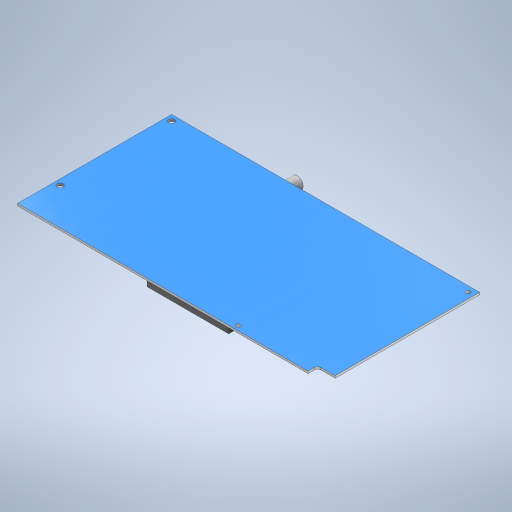
# Autodesk Inventor part: motherboard
Saved by Autodesk Inventor 2024 (Build 280153000, 153)
## iProperties
Created: 2024-09-23
Part Number: motherboard
Material: Generic
Document SubType Name: Modeling
Designer: PC
Density: 1 g/cm^3
Appearance: Default
Author: PC
Autodesk Inventor part; units mm, degrees
ref_plane "YZ Plane" through (0, 0, 0) normal (1, 0, 0) x (0, 1, 0)
ref_plane "XZ Plane" through (0, 0, 0) normal (0, 1, 0) x (-1, 0, 0)
ref_plane "XY Plane" through (0, 0, 0) normal (0, 0, 1) x (1, 0, 0)
sketch "Sketch1" plane through (0, 0, 0) normal (0, 1, 0) x (-1, 0, 0)
  line L0 (12, 0) -> (210, 0)
  line L1 (210, 0) -> (210, -105)
  line L2 (210, -105) -> (0, -105)
  circle A0 centre (4, -101) radius 1.5
  circle A1 centre (206, -101) radius 2
  circle A2 centre (206, -25) radius 2
  circle A3 centre (62.6, -3) radius 1.5
  line L3 (12, 0) -> (12, -4.5)
  line L4 (10, -6.5) -> (0, -6.5)
  arc A4 (10, -6.5) -> (12, -4.5) centre (10, -4.5) ccw
  line L5 (0, -6.5) -> (0, -105)
  point P0 (0, 0)
  point P1 (12, -6.5)
  dimension "d0" = 105
  dimension "d1" = 210
  dimension "d4" = 4
  dimension "d6" = 3
  dimension "d7" = 4
  dimension "d8" = 4
  dimension "d9" = 4
  dimension "d10" = 76
  dimension "d12" = 3
  dimension "d13" = 3
  dimension "d14" = 12
  dimension "d15" = 6.5
  dimension "d16" = 2
  constraints: 12 end point, 5 centre point, 2 point on circle, 2 point on line, 2 tangent, 1 horizontal, 1 parallel, 1 perpendicular, 1 vertical
  measures "d0" distance of L0.end L1.end
  measures "d1" distance of L1.end L2.end
  measures "d4" distance from line of L2 A0.centre
  measures "d6" diameter of A0
  measures "d7" diameter of A1
  measures "d8" distance from line of L1 A1.centre
  measures "d9" diameter of A2
  measures "d10" distance of A1.centre A2.centre
  measures "d12" distance from line of L0 A3.centre
  measures "d13" diameter of A3
  measures "d14" distance of point (12, -6.5) L4.end
  measures "d15" distance of L0.start point (12, -6.5)
  measures "d16" radius of A4
extrude "Extrusion1" add sketch "Sketch1" along normal blind 1.5
sketch "Sketch2" plane through (0, 0, 0) normal (0, -1, 0) x (1, 0, 0)
  line L0 (-126.75, -5) -> (-71.15, -5)
  line L1 (-71.15, -5) -> (-71.15, -9.5)
  line L2 (-71.15, -9.5) -> (-126.75, -9.5)
  line L3 (-126.75, -9.5) -> (-126.75, -5)
  line L4 (-210, -105) -> (-210, 0) projected
  line L5 (0, -6.5) -> (0, -105) projected
  line L6 (-72.7, -8.25) -> (-125.2, -8.25)
  line L7 (-125.2, -8.25) -> (-125.2, -6.25)
  line L8 (-125.2, -6.25) -> (-72.7, -6.25)
  line L9 (-72.7, -6.25) -> (-72.7, -8.25)
  line L10 (-210, 0) -> (-12, 0) projected
  point P0 (0, 0)
  point P1 (-126.75, -7.25)
  point P2 (-72.7, -7.25)
  point P3 (-71.15, -7.25)
  point P4 (-98.95, -6.25)
  point P5 (-98.95, -5)
  point P6 (-111, 0)
  dimension "d17" = 4.5
  dimension "d18" = 55.6
  dimension "d33" = 52.5
  dimension "d34" = 2
  dimension "d35" = 71.15
  dimension "d36" = 5
  constraints: 16 end point, 6 midpoint, 4 parallel, 2 horizontal, 2 perpendicular, 1 horizontal alignment, 1 vertical alignment
  measures "d17" distance between parallel lines of L2 L0
  measures "d18" distance of L1.end L2.end
  measures "d33" distance of L6.start L6.end
  measures "d34" distance between parallel lines of L8 L6
  measures "d35" distance from line of L5 L0.end
  measures "d36" distance from line of point (-111, 0) L0
sketch "Sketch3" plane through (0, 0, 0) normal (0, -1, 0) x (1, 0, 0)
  line L0 (0, -105) -> (-210, -105) projected
  line L1 (-55.6, -105) -> (-86.6, -105)
  line L2 (-86.6, -105) -> (-86.6, -89)
  line L3 (-86.6, -89) -> (-55.6, -89)
  line L4 (-55.6, -89) -> (-55.6, -105)
  line L5 (0, -6.5) -> (0, -105) projected
  point P0 (0, 0)
  point P1 (-55.6, -97)
  dimension "d23" = 55.6
  dimension "d24" = 31
  dimension "d25" = 16
  constraints: 8 end point, 2 parallel, 1 horizontal, 1 midpoint, 1 perpendicular, 1 point on line
  measures "d23" distance from line of L5 point (-55.6, -97)
  measures "d24" distance of L2.end L3.end
  measures "d25" distance of L1.end L2.end
extrude "Extrusion3" add sketch "Sketch3" along normal blind 12.5
sketch "Sketch4" plane through (0, 0, 0) normal (0, -1, 0) x (1, 0, 0)
  line L0 (-2.4, -105) -> (-210, -105)
  line L1 (-105, -105) -> (-120.2, -105)
  line L2 (-120.2, -105) -> (-120.2, -92.25)
  line L3 (-120.2, -92.25) -> (-106.2, -92.25)
  line L4 (-106.2, -92.25) -> (-106.2, -105)
  line L5 (-86.6, -89) -> (-86.6, -105) projected
  point P0 (0, 0)
  point P1 (-120.2, -105)
  dimension "d28" = 12.75
  dimension "d29" = 14
  dimension "d32" = 19.6
  constraints: 10 end point, 2 parallel, 1 horizontal, 1 midpoint, 1 perpendicular
  measures "d28" distance of L1.end L2.end
  measures "d29" distance of L2.end L3.end
  measures "d32" distance between parallel lines of L5 L4
extrude "Extrusion4" add sketch "Sketch4" along normal blind 13.15
extrude "Extrusion5" add sketch "Sketch2" along normal blind 8.6
sketch "Sketch5" plane through (0, 0, 0) normal (0, -1, 0) x (1, 0, 0)
  line L0 (0, -105) -> (-210, -105) projected
  line L1 (-185, -105) -> (-173.5, -105)
  line L2 (-173.5, -105) -> (-173.5, -88)
  line L3 (-173.5, -88) -> (-185, -88)
  line L4 (-185, -88) -> (-185, -105)
  line L5 (-210, -105) -> (-210, 0) projected
  point P0 (0, 0)
  dimension "d39" = 17
  dimension "d40" = 11.5
  dimension "d43" = 25
  constraints: 8 end point, 2 parallel, 1 horizontal, 1 perpendicular, 1 point on line
  measures "d39" distance of L3.end L1.start
  measures "d40" distance of L2.end L3.end
  measures "d43" distance between parallel lines of L5 L4
extrude "Extrusion6" add sketch "Sketch5" along normal blind 11
sketch "Sketch6" plane through (0, 0, 0) normal (0, -1, 0) x (1, 0, 0)
  line L0 (0, -105) -> (-210, -105) projected
  line L1 (-139.4357, -105) -> (-129.4357, -105)
  line L2 (-129.4357, -105) -> (-129.4357, -95)
  line L3 (-129.4357, -95) -> (-139.4357, -95)
  line L4 (-139.4357, -95) -> (-139.4357, -105)
  point P0 (0, 0)
  dimension "d44" = 10
  dimension "d45" = 10
  constraints: 8 end point, 2 parallel, 1 horizontal, 1 perpendicular, 1 point on line
  measures "d44" distance of L2.end L3.end
  measures "d45" distance of L3.end L1.start
extrude "Extrusion7" add sketch "Sketch6" along normal blind 12
sketch "Sketch7" plane through (0, 1.5, -105) normal (0, 0, -1) x (-1, 0, 0)
  circle A0 centre (134.4357, -7.5) radius 4.15
  line L0 (139.4357, -1.5) -> (139.4357, -13.5) projected
  line L1 (139.4357, -13.5) -> (129.4357, -13.5) projected
  point P0 (0, -1.5)
  point P1 (139.4357, -7.5)
  point P2 (134.4357, -13.5)
  dimension "d48" = 8.3
  constraints: 2 midpoint, 1 centre point, 1 horizontal alignment, 1 vertical alignment
  measures "d48" diameter of A0
extrude "Extrusion8" add sketch "Sketch7" along normal blind 10
body "Solid1"
